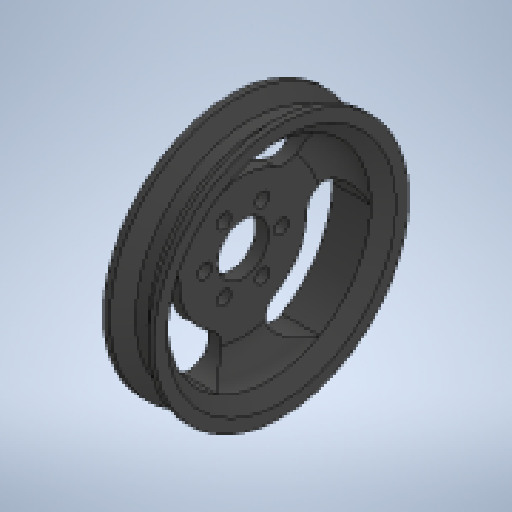
# Autodesk Inventor part: Temp - Wheel
Saved by Autodesk Inventor 2023.2 (Build 272271000, 271)
## iProperties
Created: 2023-06-26
Part Number: Temp - Wheel
Material: Nylon 6/6
Document SubType Name: Modeling
Designer: Nathan Cai
Density: 1.13 g/cm^3
Appearance: Rubber - Black
Mass: 15.2385 g
Surface Area: 93.3567 cm^2
Volume: 13.4854 cm^3
Author: Nathan Cai
Autodesk Inventor part; units mm, degrees
ref_plane "YZ Plane" through (0, 0, 0) normal (1, 0, 0) x (0, 1, 0)
ref_plane "XZ Plane" through (0, 0, 0) normal (0, 1, 0) x (-1, 0, 0)
ref_plane "XY Plane" through (0, 0, 0) normal (0, 0, 1) x (1, 0, 0)
sketch "Sketch1" plane through (0, 0, 0) normal (1, 0, 0) x (0, 1, 0)
  circle A0 centre (0, 0) radius 31.75
  circle A1 centre (0, 0) radius 9.525 construction
  circle A2 centre (0, 0) radius 6.35
  line L0 (0, 9.525) -> (0, 0) construction
  circle A3 centre (0, 9.525) radius 1.7526
  circle A4 centre (-8.248892, 4.7625) radius 1.7526
  circle A5 centre (-8.248892, -4.7625) radius 1.7526
  circle A6 centre (0, -9.525) radius 1.7526
  circle A7 centre (8.248892, -4.7625) radius 1.7526
  circle A8 centre (8.248892, 4.7625) radius 1.7526
  circle A9 centre (0, 0) radius 25.4
  line L1 (0, 0) -> (0, -25.4) construction
  arc A10 (-17.872599, -10.31875) -> (0, -20.6375) centre (0, 0) ccw construction
  arc A11 (-21.997045, -12.7) -> (0, -25.4) centre (0, 0) ccw
  arc A12 (-13.748153, -7.9375) -> (0, -15.875) centre (0, 0) ccw
  arc A13 (-13.748153, -7.9375) -> (-21.997045, -12.7) centre (-17.872599, -10.31875) ccw
  arc A14 (0, -25.4) -> (0, -15.875) centre (0, -20.6375) ccw
  line L2 (0, 0) -> (-17.872599, -10.31875) construction
  line L3 (0, 0) -> (0, -20.6375) construction
  arc A15 (21.997045, 12.7) -> (13.748153, 7.9375) centre (17.872599, 10.31875) ccw
  arc A16 (13.748153, -7.9375) -> (21.997045, -12.7) centre (17.872599, -10.31875) ccw
  arc A17 (13.748153, -7.9375) -> (13.748153, 7.9375) centre (0, 0) ccw
  arc A18 (17.872599, -10.31875) -> (17.872599, 10.31875) centre (0, 0) ccw construction
  arc A19 (21.997045, -12.7) -> (21.997045, 12.7) centre (0, 0) ccw
  arc A20 (-21.997045, 12.7) -> (-13.748153, 7.9375) centre (-17.872599, 10.31875) ccw
  arc A21 (0, 15.875) -> (0, 25.4) centre (0, 20.6375) ccw
  arc A22 (0, 15.875) -> (-13.748153, 7.9375) centre (0, 0) ccw
  arc A23 (0, 20.6375) -> (-17.872599, 10.31875) centre (0, 0) ccw construction
  arc A24 (0, 25.4) -> (-21.997045, 12.7) centre (0, 0) ccw
  point P0 (8.687312, -23.868193)
  point P1 (8.248892, -4.7625)
  point P2 (8.248892, 4.7625)
  point P3 (0, 9.525)
  point P4 (-8.248892, 4.7625)
  point P5 (0, 25.4)
  point P6 (-21.997045, 12.7)
  point P7 (-21.997045, -12.7)
  point P8 (21.997045, -12.7)
  dimension "d3" = 19.05
  dimension "d0" = 63.5
  dimension "d4" = 12.7
  dimension "d5" = 3.5052
  dimension "d8" = 360
  dimension "d10" = 50.8
  dimension "d20" = 60
  dimension "d21" = 9.525
  dimension "d24" = 360
  constraints: 33 point on circle, 24 centre point, 8 end point, 7 coincident, 4 tangent, 2 vertical, 1 point on line, 1 vertical alignment, 61 other
  measures "d0" diameter of A0
  measures "d4" diameter of A2
  measures "d5" diameter of A3
  measures "d10" diameter of A9
  measures "d20" angle of L2 L3
  measures "d21" diameter of A13
extrude "Extrusion1" add sketch "Sketch1" along normal blind 12.7 contours A0 | A15 A17 A16 A9 A14 A12 A13 A20 A22 A21
sketch "Sketch2" plane through (12.7, 0, 0) normal (1, 0, 0) x (0, 0, -1)
  circle A0 centre (0, 0) radius 6.35 projected
  circle A1 centre (0, 0) radius 25.4
  point P0 (-12.7, 21.997045)
  constraints: 1 coincident, 3 other
extrude "Extrusion2" cut sketch "Sketch2" against normal blind 9.525 contours A0 | A1
fillet "Fillet1" radius 6.35 3 edges at (3.175, -25.4, 0) (3.175, 12.7, 21.997) (3.175, 12.7, -21.997)
sketch "Sketch3" plane through (0, 0, 0) normal (0, 1, 0) x (-1, 0, 0)
  line L0 (-11.1125, -28.575) -> (-1.5875, -28.575)
  line L1 (-1.5875, -28.575) -> (-1.5875, -34.925)
  line L2 (-1.5875, -34.925) -> (-11.1125, -34.925)
  line L3 (-11.1125, -34.925) -> (-11.1125, -28.575)
  line L4 (0, -31.75) -> (-12.7, -31.75) projected
  line L5 (-11.1125, -28.575) -> (-1.5875, -34.925) construction
  line L6 (-1.5875, -28.575) -> (-11.1125, -34.925) construction
  line L7 (0, 0) -> (-12.7, 0) construction
  line L8 (-12.7, 31.75) -> (-12.7, -31.75) projected
  point P0 (-6.35, -31.75)
  point P1 (-1.5875, -31.75)
  point P2 (-11.1125, -31.75)
  dimension "d26" = 9.525
  dimension "d27" = 6.35
  constraints: 14 end point, 4 midpoint, 2 parallel, 1 horizontal, 1 perpendicular
  measures "d26" distance of L1.end L2.end
  measures "d27" distance of L0.end L1.end
revolve "Revolution1" cut sketch "Sketch3" angle 360 about axis through (0, 0, 0) along (1, 0, 0)
chamfer "Chamfer1" distance 3.175 angle 45 2 edges at (11.1125, 0, 28.575) (1.5875, 0, 28.575)
chamfer "Chamfer2" distance 3.175 angle 45 6 edges at (12.7, -12.7, -21.997) (12.7, 25.4, 0) (12.7, -12.7, 21.997) (12.7, -25.4, 0) (12.7, 12.7, 21.997) (12.7, 12.7, -21.997)
body "Solid1"
